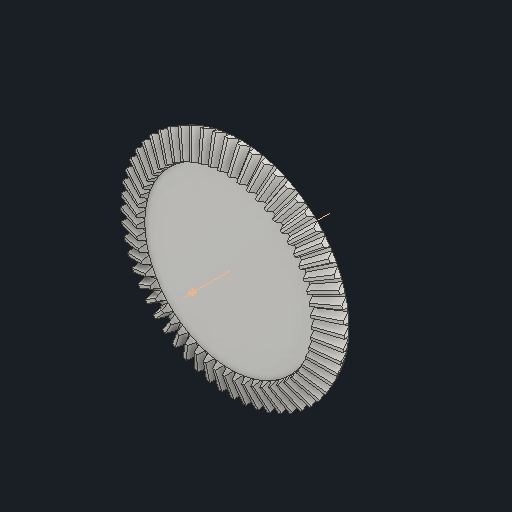
# Autodesk Inventor part: Bevel Gear2
Saved by Autodesk Inventor 2027.1 (Build 311267000, 267)
## iProperties
Created: 2026-10-02
Part Number: Bevel Gear2
Material: Steel, Mild
Document SubType Name: Modeling
Designer: HP
Categories: <?xml version="1.0" encoding="UTF-16"?> <MemberInstance><Categories><FamilyTemplate><FamilyTemplateParameter ValueType="xs:double" Id="1" ObjectReferenceKey="da_z" ObjectType="kUserParameterObject"/><FamilyTemplateParameter ValueType="xs:double" Id="2" ObjectReferenceKey="da_b" ObjectType="kUserParameterObject"/><FamilyTemplateParameter ValueType="xs:double" Id="3" ObjectReferenceKey="da_beta" ObjectType="kUserParameterObject"/><FamilyTemplateParameter ValueType="xs:double" Id="4" ObjectReferenceKey="da_dae" ObjectType="kUserParameterObject"/><FamilyTemplateParameter ValueType="xs:double" Id="5" ObjectReferenceKey="da_ve" ObjectType="kUserParameterObject"/><FamilyTemplateParameter ValueType="xs:double" Id="6" ObjectReferenceKey="da_omega" ObjectType="kUserParameterObject"/><FamilyTemplateParameter ValueType="xs:string" Id="7" ObjectReferenceKey="EAIAABAAAAAAHwAAAAAAAIAAAAAAAAAA" ObjectType="83914240" SubObjectId="SurfaceGeometry"/></FamilyTemplate><ParamToTemplateMap><ParamToTemplate CategoryParameter="//CategoryParameter[@InternalName='046C89C9-8512-4d59-83FE-43B91F4F132A']" TemplateParameter="1"/><ParamToTemplate CategoryParameter="//CategoryParameter[@InternalName='2552DF32-E462-4b46-AEBF-C6C7768E72AC']" TemplateParameter="2"/><ParamToTemplate CategoryParameter="//CategoryParameter[@InternalName='C9EE641D-15FC-4fae-A226-E94C4372FDD7']" TemplateParameter="3"/><ParamToTemplate><ParamToTemplate CategoryParameter="//CategoryParameter[@InternalName='00B6519A-459B-49c7-AD84-2E56D39A5744']" ConstantValue="-0.000000"/></ParamToTemplate><ParamToTemplate><ParamToTemplate CategoryParameter="//CategoryParameter[@InternalName='04B31F0E-C7A6-4894-AA32-9629BEFACF47']" ConstantValue="1.000000"/></ParamToTemplate><ParamToTemplate><ParamToTemplate CategoryParameter="//CategoryParameter[@InternalName='43CBEC2E-7847-49e7-A936-2F7889FCB2D9']" ConstantValue="0.200000"/></ParamToTemplate><ParamToTemplate><ParamToTemplate CategoryParameter="//CategoryParameter[@InternalName='B1EFC894-105D-4ebd-86BF-FA20ED196853']" ConstantValue="0.300000"/></ParamToTemplate><ParamToTemplate><ParamToTemplate CategoryParameter="//CategoryParameter[@InternalName='51175063-3D10-4879-93E8-6246FE8B403D']" ConstantValue="2060000000.000000"/></ParamToTemplate><ParamToTemplate><ParamToTemplate CategoryParameter="//CategoryParameter[@InternalName='A3A52E27-4454-46a9-B0BD-C932399B70AF']" ConstantValue="0.300000"/></ParamToTemplate><ParamToTemplate CategoryParameter="//CategoryParameter[@InternalName='2A200944-5A8C-41ca-B96E-8520D2E510F1']" TemplateParameter="4"/><ParamToTemplate><ParamToTemplate CategoryParameter="//CategoryParameter[@InternalName='1A637F62-92C8-44bc-B81F-10802510B579']" ConstantValue="13.566412"/></ParamToTemplate><ParamToTemplate CategoryParameter="//CategoryParameter[@InternalName='B52DD4BE-6863-48fb-BF58-89EF6F9EC65C']" TemplateParameter="5"/><ParamToTemplate><ParamToTemplate CategoryParameter="//CategoryParameter[@InternalName='3956BFF2-84D2-457d-93C2-9B0613DEBA67']" ConstantValue="2.483756"/></ParamToTemplate><ParamToTemplate CategoryParameter="//CategoryParameter[@InternalName='739CFA02-461B-4bf8-8049-181FCAD8B28F']" TemplateParameter="6"/><ParamToTemplate><ParamToTemplate CategoryParameter="//CategoryParameter[@InternalName='A27E999F-E2CE-4481-8A2A-EBF499C4C3C5']" ConstantValue="-0.000000"/></ParamToTemplate><ParamToTemplate><ParamToTemplate CategoryParameter="//CategoryParameter[@InternalName='9E1B4470-B2D3-4ff1-B813-535BB4CDF51A']" ConstantValue="3520000.000000"/></ParamToTemplate><ParamToTemplate><ParamToTemplate CategoryParameter="//CategoryParameter[@InternalName='F8452263-BFF6-458c-9FB1-07C4B99E95CD']" ConstantValue="11400000.000000"/></ParamToTemplate><ParamToTemplate><ParamToTemplate CategoryParameter="//CategoryParameter[@InternalName='3E3BB259-FD49-497f-8171-6EBC954A3479']" ConstantValue="2.000000"/></ParamToTemplate><ParamToTemplate CategoryParameter="//CategoryParameter[@InternalName='27C3BAF2-7550-4e4b-AE2C-0DB134B7D9B7']" TemplateParameter="7"/></ParamToTemplateMap><Category DisplayName="Gear" InternalName="DC85795E-93AB-48d5-8EEE-5A27447B64BD" Mnemonic="Gear"><CategoryParameter DisplayName="z" InternalName="046C89C9-8512-4d59-83FE-43B91F4F132A" Mnemonic="z"/><CategoryParameter DisplayName="b" InternalName="2552DF32-E462-4b46-AEBF-C6C7768E72AC" Mnemonic="b"/><CategoryParameter DisplayName="||b|" InternalName="C9EE641D-15FC-4fae-A226-E94C4372FDD7" Mnemonic="beta"/><CategoryParameter DisplayName="x" InternalName="00B6519A-459B-49c7-AD84-2E56D39A5744" Mnemonic="x"/><CategoryParameter DisplayName="a*" InternalName="04B31F0E-C7A6-4894-AA32-9629BEFACF47" Mnemonic="a"/><CategoryParameter DisplayName="c*" InternalName="43CBEC2E-7847-49e7-A936-2F7889FCB2D9" Mnemonic="c"/><CategoryParameter DisplayName="r|.f|*" InternalName="B1EFC894-105D-4ebd-86BF-FA20ED196853" Mnemonic="rf"/><CategoryParameter DisplayName="E" InternalName="51175063-3D10-4879-93E8-6246FE8B403D" Mnemonic="E"/><CategoryParameter DisplayName="||m|" InternalName="A3A52E27-4454-46a9-B0BD-C932399B70AF" Mnemonic="mi"/><Category DisplayName="BevelGear" InternalName="0C98F69A-0C2B-4791-B2FE-7691BB227E77" Mnemonic="BevelGear"><CategoryParameter DisplayName="d|.ae|" InternalName="2A200944-5A8C-41ca-B96E-8520D2E510F1" Mnemonic="dae"/><CategoryParameter DisplayName="d|.ai|" InternalName="1A637F62-92C8-44bc-B81F-10802510B579" Mnemonic="dai"/><CategoryParameter DisplayName="A|.e|" InternalName="B52DD4BE-6863-48fb-BF58-89EF6F9EC65C" Mnemonic="ve"/><CategoryParameter DisplayName="A|.i|" InternalName="3956BFF2-84D2-457d-93C2-9B0613DEBA67" Mnemonic="vi"/><CategoryParameter DisplayName="||S|" InternalName="739CFA02-461B-4bf8-8049-181FCAD8B28F" Mnemonic="omega"/><CategoryParameter DisplayName="x|.t|" InternalName="A27E999F-E2CE-4481-8A2A-EBF499C4C3C5" Mnemonic="xt"/><CategoryParameter DisplayName="||s||.Flim|" InternalName="9E1B4470-B2D3-4ff1-B813-535BB4CDF51A" Mnemonic="sFlim"/><CategoryParameter DisplayName="||s||.Hlim|" InternalName="F8452263-BFF6-458c-9FB1-07C4B99E95CD" Mnemonic="sHlim"/><CategoryParameter DisplayName="type" InternalName="3E3BB259-FD49-497f-8171-6EBC954A3479" Mnemonic="type"/><CategoryParameter DisplayName="PitchDiameter" InternalName="27C3BAF2-7550-4e4b-AE2C-0DB134B7D9B7" Mnemonic="IDS_PITCHDIAM"/></Category></Category></Categories></MemberInstance>
Mass: 60.9118 g
Surface Area: 34.3074 cm^2
Volume: 7.7496 cm^3
Density: 7.86 g/cm^3
Appearance: Steel
CustomPartVersion: 1
Author: HP
Autodesk Inventor part; units mm, degrees
ref_plane "Mesh Plane2" through (0, 0, 0) normal (0.9984815, 0.0550878, 0) x (0, 0, 1)
sketch "Teeth Body Sketch" plane through (0, 0, 0) normal (1, 0, 0) x (0, 1, 0)
  line L0 (0, 0) -> (84.152901, -37.838462) construction
  line L1 (84.152901, -37.838462) -> (86.622582, -31.717949)
  line L2 (86.622582, -31.717949) -> (0, 0) construction
  line L3 (85.5, -34.5) -> (0, 0) construction
  line L4 (65.898111, -29.630388) -> (67.832058, -24.837562)
  line L5 (84.152901, -37.838462) -> (65.898111, -29.630388)
  line L6 (86.622582, -31.717949) -> (67.832058, -24.837562)
  line L7 (0, -39.386751) -> (0, 6.564458)
  line L8 (0, -34.5) -> (86.622582, -34.5) construction
  dimension "d0" = 171
  dimension "d1" = 168.3058
  dimension "d2" = 173.24516
  dimension "d3" = 20
  dimension "d4" = 31.71795
  constraints: 16 end point, 4 point on line, 3 perpendicular, 2 collinear, 1 horizontal alignment, 1 vertical alignment
  measures "d0" diameter of L3.start L7
  measures "d1" diameter of L0.end L7
  measures "d2" diameter of L1.end L7
  measures "d3" distance between parallel lines of L1 L4
  measures "d4" vertical distance of L1.end L0.start
revolve "Teeth Body" add sketch "Teeth Body Sketch" angle 360 about axis through (0, 0, 0) along (0, 0, 1)
ref_plane "Tooth Plane" through (0, 85.5, -34.5) normal (0, -0.9273504, 0.374194) x (1, 0, 0)
sketch "Start Sketch" plane through (0, 85.5, -34.5) normal (0, -0.9273504, 0.374194) x (1, 0, 0)
  line L0 (0, -23.505131) -> (0, 10.644758)
  arc A0 (-0.944442, -4.392) -> (-4.360141, 4.939283) centre (-76.874908, -26.895415) ccw
  arc A1 (4.360141, 4.939283) -> (0.944442, -4.392) centre (76.874908, -26.895415) ccw
  line L1 (-0.944442, -4.392) -> (0.944442, -4.392)
  arc A2 (4.360141, 4.939283) -> (-4.360141, 4.939283) centre (0, -228.491083) ccw
  dimension "d7" = 79.19495
  dimension "d8" = 76.87491
  dimension "d9" = 201.59567
  dimension "d57" = 233.47108
  dimension "d58" = 224.09908
  constraints: 6 point on circle, 3 centre point, 3 symmetric about line, 2 end point, 1 coincident, 1 perpendicular, 1 other
  measures "d7" radius of A0
  measures "d8" horizontal distance of point (0, -228.491) A0.centre
  measures "d9" vertical distance of point (0, -228.491) A0.centre
  measures "d57" radius of A2
  measures "d58" distance from line of A2.centre L1
sketch "End Sketch" plane through (0, 66.646966, -26.892635) normal (0, -0.9273504, 0.374194) x (1, 0, 0)
  line L0 (0, -15.35404) -> (0, 6.953444)
  arc A0 (-0.736189, -3.423549) -> (-3.398715, 3.850155) centre (-59.923736, -20.964887) ccw
  arc A1 (3.398715, 3.850155) -> (0.736189, -3.423549) centre (59.923736, -20.964887) ccw
  line L1 (-0.736189, -3.423549) -> (0.736189, -3.423549)
  arc A2 (3.398715, 3.850155) -> (-3.398715, 3.850155) centre (0, -178.108039) ccw
  dimension "d12" = 61.7322
  dimension "d15" = 59.92374
  dimension "d16" = 157.14315
  dimension "d59" = 181.98993
  dimension "d60" = 174.68449
  constraints: 6 point on circle, 3 centre point, 3 symmetric about line, 2 end point, 1 coincident, 1 other
  measures "d12" radius of A0
  measures "d15" horizontal distance of A0.centre point (0, -178.108)
  measures "d16" vertical distance of A0.centre point (0, -178.108)
  measures "d59" radius of A2
  measures "d60" distance from line of A2.centre L1
loft "Loft" cut profiles "Start Sketch", "End Sketch"
pattern_circular "Circular Pattern" count 57 over 360 about axis through (0, 0, 0) along (0, 0, 1) of "Loft"
ref_plane "End Plane" through (0, 66.646966, -26.892635) normal (0, -0.9273504, 0.374194) x (1, 0, 0)
sketch3d "3D Sketch Right"
ref_plane "End Plane Right" through (-6.459448, 66.333201, -26.892635) normal (0.0898791, -0.9229846, 0.374194) x (0.9952921, 0.0969204, 0)
sketch "End Sketch Right" plane through (-6.459448, 66.333201, -26.892635) normal (0.0898791, -0.9229846, 0.374194) x (0.9952921, 0.0969204, 0)
  arc A0 (-0.736189, -3.423549) -> (-3.398715, 3.850155) centre (-59.923736, -20.964887) ccw
  line L0 (0, -215.148877) -> (0, 40.807493)
  arc A1 (3.398715, 3.850155) -> (0.736189, -3.423549) centre (59.923736, -20.964887) ccw
  line L1 (-0.736189, -3.423549) -> (0.736189, -3.423549)
  arc A2 (3.398715, 3.850155) -> (-3.398715, 3.850155) centre (0, -178.108039) ccw
  dimension "d70" = 59.92374
  dimension "d71" = 157.14315
  dimension "d72" = 61.7322
  dimension "d73" = 174.68449
  dimension "d74" = 181.98993
  constraints: 6 point on circle, 3 centre point, 3 symmetric about line, 2 end point, 1 coincident, 1 perpendicular, 1 other
  measures "d70" horizontal distance of A2.centre A0.centre
  measures "d71" vertical distance of point (0, -178.108) A0.centre
  measures "d72" radius of A0
  measures "d73" distance from line of point (0, -178.108) L1
  measures "d74" radius of A2
feature "Loft Right" [suppressed]
pattern_circular "Circular Pattern Right" [suppressed]
sketch3d "3D Sketch Left"
ref_plane "End Plane Left" through (6.513752, 66.333201, -26.939081) normal (-0.0906066, -0.9226984, 0.3747241) x (0.9952132, -0.0977274, 0)
sketch "End Sketch Left" plane through (6.513752, 66.333201, -26.939081) normal (-0.0906066, -0.9226984, 0.3747241) x (0.9952132, -0.0977274, 0)
  line L0 (0, -215.775939) -> (0, 41.477971)
  arc A0 (-0.736189, -3.382439) -> (-3.398715, 3.891265) centre (-59.923736, -20.923776) ccw
  arc A1 (3.398715, 3.891265) -> (0.736189, -3.382439) centre (59.923736, -20.923776) ccw
  line L1 (-0.736189, -3.382439) -> (0.736189, -3.382439)
  ellipse E0 centre (0, -23.027807) end of major axis (67.832058, -23.027807) minor radius 25.418305
  arc A2 (3.398715, 3.891265) -> (-3.398715, 3.891265) centre (0, -178.066929) ccw
  dimension "d56" = 25.4183
  dimension "d30" = 61.7322
  dimension "d31" = 59.92374
  dimension "d32" = 157.14315
  dimension "d61" = 181.98993
  dimension "d62" = 174.68449
  constraints: 6 point on circle, 3 centre point, 3 symmetric about line, 2 end point, 1 coincident, 2 other
  measures "d30" radius of A0
  measures "d31" horizontal distance of point (0, -178.067) A0.centre
  measures "d32" vertical distance of A0.centre point (0, -178.067)
  measures "d61" radius of A2
  measures "d62" distance from line of point (0, -178.067) L1
feature "Loft Left" [suppressed]
pattern_circular "Circular Pattern Left" [suppressed]
sketch "Body Sketch" plane through (0, 0, 0) normal (1, 0, 0) x (0, 1, 0)
  line L0 (0, -35.037536) -> (0, -19.530831)
  line L1 (84.152901, -37.838462) -> (65.898111, -29.630388)
  line L2 (65.898111, -29.630388) -> (0, -29.630388)
  line L3 (84.152901, -37.838462) -> (0, -37.838462)
  constraints: 4 end point, 2 perpendicular, 2 point on line
sketch "Body Sketch outline for Fix Body" plane through (0, 0, 0) normal (1, 0, 0) x (0, 1, 0)
  line L0 (0, -37.838462) -> (84.152901, -37.838462)
  line L1 (0, -29.630388) -> (0, -37.838462)
  line L2 (65.898111, -29.630388) -> (0, -29.630388)
  line L3 (84.152901, -37.838462) -> (65.898111, -29.630388)
revolve "Fix Body" add sketch "Body Sketch outline for Fix Body" angle 360 about axis through (0, 0, 0) along (0, 0, 1)
sketch "Sketch6" plane through (0, 0, 0) normal (1, 0, 0) x (0, 1, 0)
  line L0 (85.5, -34.5) -> (0, 0)
  line L1 (0, -37.799919) -> (0, 6.299986)
surface revolve "Pitch Diameter" sketch "Sketch6" angle 360 about axis through (0, 0, 0) along (0, 0, 1) shown no curves L0
equation "\"d0\" = da_de"
equation "\"d1\" = da_dfe"
equation "\"d2\" = da_dae"
equation "\"d3\" = da_b"
equation "\"d4\" = da_ve"
equation "\"d7\" = fd_rr"
equation "\"d8\" = fd_x"
equation "\"d9\" = fd_y"
equation "\"d57\" = 0.5 * fd_dva + 0.3 * da_he"
equation "\"d58\" = 0.5 * fd_dva - 1.12 * da_he"
equation "\"da_teethtype\" = 0"
equation "\"da_b\" = 20"
equation "\"da_de\" = 171"
equation "\"da_dae\" = 173.24516"
equation "\"da_dfe\" = 168.3058"
equation "\"da_le\" = 92.19816"
equation "\"da_omega\" = 90deg"
equation "\"da_beta\" = 0"
equation "\"da_delta\" = 68.025492deg"
equation "\"da_alpha\" = 20deg"
equation "\"da_he\" = 6.6"
equation "\"da_ve\" = 31.71795"
equation "\"da_zv\" = 152.327388"
equation "\"fd_loft\" = da_b + 0.05 * da_he"
equation "\"fd_x\" = fd_x1 + fd_x2"
equation "\"fd_y\" = fd_y1 - fd_y2"
equation "\"fd_dd\" = fd_dva - 0.8 * da_he"
equation "\"da_dvw\" = 456.98217"
equation "\"d11\" = fd_loft"
equation "\"da_dm\" = 152.45299"
equation "\"da_x\" = 0"
equation "\"da_m\" = 3"
equation "\"d50\" = da_omega"
equation "\"fd_rr\" = 79.194946"
equation "\"fd_dva\" = 462.982165"
equation "\"fd_x1\" = 2.382331"
equation "\"fd_x2\" = 74.492577"
equation "\"fd_y1\" = 228.478663"
equation "\"fd_y2\" = 26.882995"
body "Solid1"
body "Srf1"
